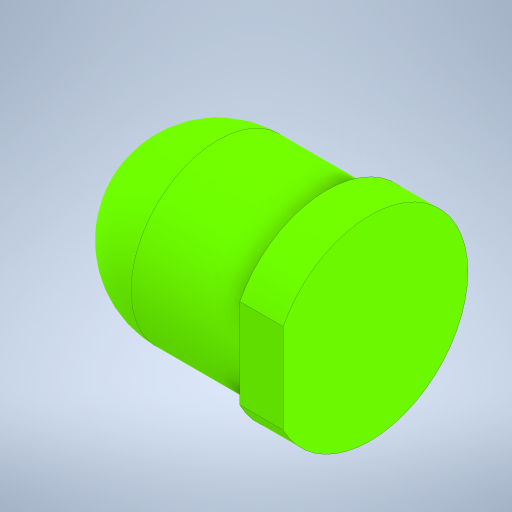
# Autodesk Inventor part: LED 8mm
Saved by Autodesk Inventor 2023 (Build 270158000, 158)
## iProperties
Created: 2022-05-21
Part Number: LED 8mm
Material: Generic
Document SubType Name: Modeling
Designer: Jochen
Density: 1 g/cm^3
Appearance: Default
Author: Jochen
Autodesk Inventor part; units mm, degrees
ref_plane "YZ Plane" through (0, 0, 0) normal (1, 0, 0) x (0, 1, 0)
ref_plane "XZ Plane" through (0, 0, 0) normal (0, 1, 0) x (-1, 0, 0)
sketch "Sketch1" plane through (0, 0, 0) normal (0, 0, 1) x (1, 0, 0)
  line L0 (0, -0.9657) -> (0, 5.7941) construction
  line L1 (-14.1941, 0) -> (2.3657, 0) construction
  line L2 (0, 4.5) -> (0, 0)
  line L3 (-7, 4) -> (-2, 4)
  line L4 (-2, 4) -> (-2, 4.5)
  line L5 (-2, 4.5) -> (0, 4.5)
  arc A0 (-7, 4) -> (-11, 0) centre (-7, 0) ccw
  line L6 (-11, 0) -> (0, 0)
  dimension "d0" = 4
  dimension "d1" = 2
  dimension "d2" = 4.5
  dimension "d3" = 11
  constraints: 10 end point, 2 collinear, 2 perpendicular, 2 point on circle, 1 centre point, 1 line through centre, 1 parallel, 1 point on line, 1 tangent
  measures "d0" radius of A0
  measures "d1" distance of L4.end L2.start
  measures "d2" distance between parallel lines of L1 L5
  measures "d3" distance of L2.end L6.start
revolve "Revolution1" add sketch "Sketch1" angle 360 about axis through (-10, 0, 0) along (1, 0, 0)
ref_plane "Work Plane2" through (0, 0, 4) normal (0, 0, 1) x (1, 0, 0)
split "Split2" plane through (0, 0, 4) removes the side toward (0, 0, 1)
body "Solid1"
